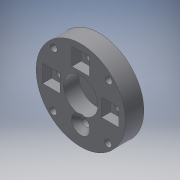
# Autodesk Inventor part: amt_socket
Saved by Autodesk Inventor 2019 (Build 230136000, 136)
## iProperties
Created: 2024-04-30
Part Number: amt_socket
Material: Generisch
Document SubType Name: Modeling
Designer: nic
Density: 1 g/cm^3
Appearance: Vorgabe
Author: nic
Autodesk Inventor part; units mm, degrees
ref_plane "YZ Plane" through (0, 0, 0) normal (1, 0, 0) x (0, 1, 0)
ref_plane "XZ Plane" through (0, 0, 0) normal (0, 1, 0) x (-1, 0, 0)
ref_plane "XY Plane" through (0, 0, 0) normal (0, 0, 1) x (1, 0, 0)
sketch "Skizze1" plane through (0, 0, 0) normal (0, 0, 1) x (1, 0, 0)
  circle A0 centre (0, 0) radius 14.5
  circle A1 centre (0, 0) radius 9.55 construction
  circle A2 centre (9.55, 0) radius 1.5
  circle A3 centre (-9.55, 0) radius 1.5
  circle A4 centre (0, 9.55) radius 1.5
  dimension "d0" = 29
  dimension "d1" = 19.1
  dimension "d2" = 3
  dimension "d3" = 3
  dimension "d4" = 3
  constraints: 5 centre point, 3 point on circle, 2 coincident
  measures "d0" diameter of A0
  measures "d1" diameter of A1
  measures "d2" diameter of A2
  measures "d3" diameter of A3
  measures "d4" diameter of A4
extrude "Extrusion1" add sketch "Skizze1" along normal blind 6
sketch "Skizze2" plane through (0, 0, 6) normal (0, 0, 1) x (1, 0, 0)
  circle A0 centre (0, 0) radius 5.6
  dimension "d7" = 11.2
  constraints: 1 centre point, 1 coincident
  measures "d7" diameter of A0
extrude "Extrusion2" cut sketch "Skizze2" against normal blind 5
sketch "Skizze3" plane through (0, 0, 1) normal (0, 0, 1) x (1, 0, 0)
  circle A0 centre (0, 0) radius 5.6 projected
  circle A1 centre (0, 0) radius 1.5
  dimension "d10" = 3
  constraints: 1 centre point, 1 coincident
  measures "d10" diameter of A1
extrude "Extrusion3" cut sketch "Skizze3" against normal through all contours A1
sketch "Skizze4" plane through (0, 0, 6) normal (0, 0, 1) x (1, 0, 0)
  circle A0 centre (0, 9.55) radius 1.5 construction
  circle A1 centre (9.55, 0) radius 1.5 construction
  circle A2 centre (-9.55, 0) radius 1.5 construction
  line L0 (-2.85, 12.4) -> (2.85, 12.4)
  line L1 (2.85, 12.4) -> (2.85, 6.7)
  line L2 (2.85, 6.7) -> (-2.85, 6.7)
  line L3 (-2.85, 6.7) -> (-2.85, 12.4)
  line L4 (-2.85, 12.4) -> (2.85, 6.7) construction
  line L5 (2.85, 12.4) -> (-2.85, 6.7) construction
  line L6 (-12.4, 2.85) -> (-6.7, 2.85)
  line L7 (-6.7, 2.85) -> (-6.7, -2.85)
  line L8 (-6.7, -2.85) -> (-12.4, -2.85)
  line L9 (-12.4, -2.85) -> (-12.4, 2.85)
  line L10 (-12.4, 2.85) -> (-6.7, -2.85) construction
  line L11 (-6.7, 2.85) -> (-12.4, -2.85) construction
  line L12 (6.7, 2.85) -> (12.4, 2.85)
  line L13 (12.4, 2.85) -> (12.4, -2.85)
  line L14 (12.4, -2.85) -> (6.7, -2.85)
  line L15 (6.7, -2.85) -> (6.7, 2.85)
  line L16 (6.7, 2.85) -> (12.4, -2.85) construction
  line L17 (12.4, 2.85) -> (6.7, -2.85) construction
  point P0 (0, 0)
  point P1 (9.55, 0)
  dimension "d13" = 5.7
  dimension "d14" = 5.7
  dimension "d15" = 5.7
  dimension "d16" = 5.7
  dimension "d17" = 5.7
  dimension "d18" = 5.7
  constraints: 36 end point, 6 midpoint, 6 parallel, 3 horizontal, 3 perpendicular
  measures "d13" distance of L1.end L2.end
  measures "d14" distance of L0.end L1.end
  measures "d15" distance of L7.end L8.end
  measures "d16" distance of L6.end L7.end
  measures "d17" distance of L13.end L14.end
  measures "d18" distance of L12.end L13.end
extrude "Extrusion4" cut sketch "Skizze4" against normal blind 3
sketch "Skizze5" plane through (0, 0, 6) normal (0, 0, 1) x (1, 0, 0)
  circle A0 centre (0, 0) radius 5.6 projected
  line L0 (0, -5.6) -> (0, -8.2) construction
  circle A1 centre (0, -8.2) radius 1.45
  dimension "d21" = 2.6
  dimension "d22" = 2.9
  constraints: 2 end point, 1 centre point, 1 coincident, 1 vertical, 1 vertical alignment, 1 other
  measures "d21" distance of L0.start L0.end
  measures "d22" diameter of A1
hole "Bohrung1" at (0, -8.2, 6) direction (0, 0, -1) diameter 2.9 end through all countersink diameter 6 countersink angle 90
sketch "Skizze6" plane through (0, 0, 6) normal (0, 0, 1) x (1, 0, 0)
  circle A0 centre (-8.8221, 9.0078) radius 2.6 construction
  circle A1 centre (-8.8221, 9.0078) radius 1.15
  circle A2 centre (-9.0078, -8.8221) radius 1.15
  circle A3 centre (8.8221, -9.0078) radius 1.15
  circle A4 centre (9.0078, 8.8221) radius 1.15
  point P0 (0, 0)
  dimension "d30" = 2.3
  dimension "d33" = 360
  constraints: 4 centre point, 1 coincident, 9 other
  measures "d30" diameter of A1
extrude "Extrusion5" cut sketch "Skizze6" against normal through all
